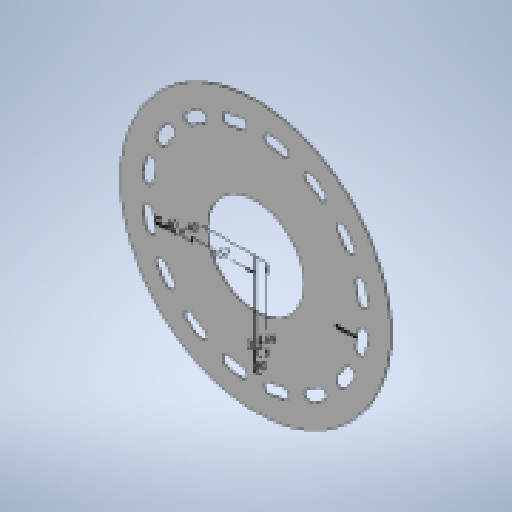
# Autodesk Inventor part: DMF 2.1 01 45 Gear ring 5
Saved by Autodesk Inventor 2026.2 (Build 302298000, 298)
## iProperties
Created: 2024-04-30
Part Number: DMF 2.1 01 45 Gear ring 5
Material: Generic
Document SubType Name: Sheet Metal
Designer: admin
Stock Number: Барабан_Сектор_Усилителя
Density: 1 g/cm^3
Sheet Metal Rule: Default
Sheet Metal Width: 0,000 mm
Sheet Metal Length: 0,000 mm
Sheet Metal Area: 0,000 mm^2
Appearance: Default
Author: pokla
Autodesk Inventor part; units mm, degrees
ref_plane "YZ Plane" through (0, 0, 0) normal (1, 0, 0) x (0, 1, 0)
ref_plane "XZ Plane" through (0, 0, 0) normal (0, 1, 0) x (-1, 0, 0)
ref_plane "XY Plane" through (0, 0, 0) normal (0, 0, 1) x (1, 0, 0)
sketch "Sketch1" plane through (0, 0, 0) normal (0, 0, 1) x (1, 0, 0)
  circle A0 centre (0, 0) radius 100
  circle A1 centre (0, 0) radius 280
  circle A2 centre (0, 0) radius 225 construction
  line L0 (-161.6581, -280) -> (-323.3162, 0)
  line L1 (-323.3162, 0) -> (-161.6581, 280)
  line L2 (-161.6581, 280) -> (161.6581, 280)
  line L3 (161.6581, 280) -> (323.3162, 0)
  line L4 (323.3162, 0) -> (161.6581, -280)
  line L5 (161.6581, -280) -> (-161.6581, -280)
  arc A3 (-28.3948, 223.2011) -> (-59.182, 217.0771) centre (0, 0) ccw construction
  arc A4 (-29.783, 234.1132) -> (-62.0754, 227.6898) centre (0, 0) ccw
  arc A5 (-27.0066, 212.2891) -> (-56.2887, 206.4645) centre (0, 0) ccw
  arc A6 (-27.0066, 212.2891) -> (-29.783, 234.1132) centre (-28.3948, 223.2011) ccw
  arc A7 (-62.0754, 227.6898) -> (-56.2887, 206.4645) centre (-59.182, 217.0771) ccw
  line L6 (-28.3948, 223.2011) -> (0, 0) construction
  line L7 (-59.182, 217.0771) -> (0, 0) construction
  line L8 (0, 0) -> (0, 100) construction
  line L9 (-43.8953, 220.6767) -> (0, 0) construction
  arc A8 (-106.1903, 185.7945) -> (-131.0145, 169.2076) centre (0, 0) ccw
  arc A9 (-106.1903, 185.7945) -> (-117.1071, 204.8949) centre (-111.6487, 195.3447) ccw
  arc A10 (-144.4833, 186.6027) -> (-131.0145, 169.2076) centre (-137.7489, 177.9052) ccw
  arc A11 (-117.1071, 204.8949) -> (-144.4833, 186.6027) centre (0, 0) ccw
  arc A12 (-111.6487, 195.3447) -> (-137.7489, 177.9052) centre (0, 0) ccw construction
  arc A13 (-169.2076, 131.0145) -> (-185.7945, 106.1903) centre (0, 0) ccw
  arc A14 (-169.2076, 131.0145) -> (-186.6027, 144.4833) centre (-177.9052, 137.7489) ccw
  arc A15 (-204.8949, 117.1071) -> (-185.7945, 106.1903) centre (-195.3447, 111.6487) ccw
  arc A16 (-186.6027, 144.4833) -> (-204.8949, 117.1071) centre (0, 0) ccw
  arc A17 (-177.9052, 137.7489) -> (-195.3447, 111.6487) centre (0, 0) ccw construction
  arc A18 (-206.4645, 56.2887) -> (-212.2891, 27.0066) centre (0, 0) ccw
  arc A19 (-206.4645, 56.2887) -> (-227.6898, 62.0754) centre (-217.0771, 59.182) ccw
  arc A20 (-234.1132, 29.783) -> (-212.2891, 27.0066) centre (-223.2011, 28.3948) ccw
  arc A21 (-227.6898, 62.0754) -> (-234.1132, 29.783) centre (0, 0) ccw
  arc A22 (-217.0771, 59.182) -> (-223.2011, 28.3948) centre (0, 0) ccw construction
  arc A23 (-212.2891, -27.0066) -> (-206.4645, -56.2887) centre (0, 0) ccw
  arc A24 (-212.2891, -27.0066) -> (-234.1132, -29.783) centre (-223.2011, -28.3948) ccw
  arc A25 (-227.6898, -62.0754) -> (-206.4645, -56.2887) centre (-217.0771, -59.182) ccw
  arc A26 (-234.1132, -29.783) -> (-227.6898, -62.0754) centre (0, 0) ccw
  arc A27 (-223.2011, -28.3948) -> (-217.0771, -59.182) centre (0, 0) ccw construction
  arc A28 (-185.7945, -106.1903) -> (-169.2076, -131.0145) centre (0, 0) ccw
  arc A29 (-185.7945, -106.1903) -> (-204.8949, -117.1071) centre (-195.3447, -111.6487) ccw
  arc A30 (-186.6027, -144.4833) -> (-169.2076, -131.0145) centre (-177.9052, -137.7489) ccw
  arc A31 (-204.8949, -117.1071) -> (-186.6027, -144.4833) centre (0, 0) ccw
  arc A32 (-195.3447, -111.6487) -> (-177.9052, -137.7489) centre (0, 0) ccw construction
  arc A33 (-131.0145, -169.2076) -> (-106.1903, -185.7945) centre (0, 0) ccw
  arc A34 (-131.0145, -169.2076) -> (-144.4833, -186.6027) centre (-137.7489, -177.9052) ccw
  arc A35 (-117.1071, -204.8949) -> (-106.1903, -185.7945) centre (-111.6487, -195.3447) ccw
  arc A36 (-144.4833, -186.6027) -> (-117.1071, -204.8949) centre (0, 0) ccw
  arc A37 (-137.7489, -177.9052) -> (-111.6487, -195.3447) centre (0, 0) ccw construction
  arc A38 (-56.2887, -206.4645) -> (-27.0066, -212.2891) centre (0, 0) ccw
  arc A39 (-56.2887, -206.4645) -> (-62.0754, -227.6898) centre (-59.182, -217.0771) ccw
  arc A40 (-29.783, -234.1132) -> (-27.0066, -212.2891) centre (-28.3948, -223.2011) ccw
  arc A41 (-62.0754, -227.6898) -> (-29.783, -234.1132) centre (0, 0) ccw
  arc A42 (-59.182, -217.0771) -> (-28.3948, -223.2011) centre (0, 0) ccw construction
  arc A43 (27.0066, -212.2891) -> (56.2887, -206.4645) centre (0, 0) ccw
  arc A44 (27.0066, -212.2891) -> (29.783, -234.1132) centre (28.3948, -223.2011) ccw
  arc A45 (62.0754, -227.6898) -> (56.2887, -206.4645) centre (59.182, -217.0771) ccw
  arc A46 (29.783, -234.1132) -> (62.0754, -227.6898) centre (0, 0) ccw
  arc A47 (28.3948, -223.2011) -> (59.182, -217.0771) centre (0, 0) ccw construction
  arc A48 (106.1903, -185.7945) -> (131.0145, -169.2076) centre (0, 0) ccw
  arc A49 (106.1903, -185.7945) -> (117.1071, -204.8949) centre (111.6487, -195.3447) ccw
  arc A50 (144.4833, -186.6027) -> (131.0145, -169.2076) centre (137.7489, -177.9052) ccw
  arc A51 (117.1071, -204.8949) -> (144.4833, -186.6027) centre (0, 0) ccw
  arc A52 (111.6487, -195.3447) -> (137.7489, -177.9052) centre (0, 0) ccw construction
  arc A53 (169.2076, -131.0145) -> (185.7945, -106.1903) centre (0, 0) ccw
  arc A54 (169.2076, -131.0145) -> (186.6027, -144.4833) centre (177.9052, -137.7489) ccw
  arc A55 (204.8949, -117.1071) -> (185.7945, -106.1903) centre (195.3447, -111.6487) ccw
  arc A56 (186.6027, -144.4833) -> (204.8949, -117.1071) centre (0, 0) ccw
  arc A57 (177.9052, -137.7489) -> (195.3447, -111.6487) centre (0, 0) ccw construction
  arc A58 (206.4645, -56.2887) -> (212.2891, -27.0066) centre (0, 0) ccw
  arc A59 (206.4645, -56.2887) -> (227.6898, -62.0754) centre (217.0771, -59.182) ccw
  arc A60 (234.1132, -29.783) -> (212.2891, -27.0066) centre (223.2011, -28.3948) ccw
  arc A61 (227.6898, -62.0754) -> (234.1132, -29.783) centre (0, 0) ccw
  arc A62 (217.0771, -59.182) -> (223.2011, -28.3948) centre (0, 0) ccw construction
  arc A63 (212.2891, 27.0066) -> (206.4645, 56.2887) centre (0, 0) ccw
  arc A64 (212.2891, 27.0066) -> (234.1132, 29.783) centre (223.2011, 28.3948) ccw
  arc A65 (227.6898, 62.0754) -> (206.4645, 56.2887) centre (217.0771, 59.182) ccw
  arc A66 (234.1132, 29.783) -> (227.6898, 62.0754) centre (0, 0) ccw
  arc A67 (223.2011, 28.3948) -> (217.0771, 59.182) centre (0, 0) ccw construction
  arc A68 (185.7945, 106.1903) -> (169.2076, 131.0145) centre (0, 0) ccw
  arc A69 (185.7945, 106.1903) -> (204.8949, 117.1071) centre (195.3447, 111.6487) ccw
  arc A70 (186.6027, 144.4833) -> (169.2076, 131.0145) centre (177.9052, 137.7489) ccw
  arc A71 (204.8949, 117.1071) -> (186.6027, 144.4833) centre (0, 0) ccw
  arc A72 (195.3447, 111.6487) -> (177.9052, 137.7489) centre (0, 0) ccw construction
  arc A73 (131.0145, 169.2076) -> (106.1903, 185.7945) centre (0, 0) ccw
  arc A74 (131.0145, 169.2076) -> (144.4833, 186.6027) centre (137.7489, 177.9052) ccw
  arc A75 (117.1071, 204.8949) -> (106.1903, 185.7945) centre (111.6487, 195.3447) ccw
  arc A76 (144.4833, 186.6027) -> (117.1071, 204.8949) centre (0, 0) ccw
  arc A77 (137.7489, 177.9052) -> (111.6487, 195.3447) centre (0, 0) ccw construction
  arc A78 (56.2887, 206.4645) -> (27.0066, 212.2891) centre (0, 0) ccw
  arc A79 (56.2887, 206.4645) -> (62.0754, 227.6898) centre (59.182, 217.0771) ccw
  arc A80 (29.783, 234.1132) -> (27.0066, 212.2891) centre (28.3948, 223.2011) ccw
  arc A81 (62.0754, 227.6898) -> (29.783, 234.1132) centre (0, 0) ccw
  arc A82 (59.182, 217.0771) -> (28.3948, 223.2011) centre (0, 0) ccw construction
  point P0 (0, -280)
  point P1 (242.4871, 140)
  point P2 (-242.4871, 140)
  point P3 (-125.0033, 187.0807)
  point P4 (-187.0807, 125.0033)
  point P5 (-220.6767, 43.8953)
  point P6 (-220.6767, -43.8953)
  point P7 (-187.0807, -125.0033)
  point P8 (-125.0033, -187.0807)
  point P9 (-43.8953, -220.6767)
  point P10 (43.8953, -220.6767)
  point P11 (125.0033, -187.0807)
  point P12 (187.0807, -125.0033)
  point P13 (220.6767, -43.8953)
  point P14 (220.6767, 43.8953)
  point P15 (187.0807, 125.0033)
  point P16 (125.0033, 187.0807)
  point P17 (43.8953, 220.6767)
  dimension "d31" = 560
  dimension "d32" = 200
  dimension "d39" = 450
  dimension "d56" = 11
  dimension "d57" = 8
  dimension "d58" = 11.25
  dimension "d61" = 360
  measures "d56" radius of A7
  measures "d57" angle of L7 L6
  measures "d58" angle of L8 L9
extrude "Plate4" add sketch "Sketch1" along normal blind 2 contours A1
sketch "Sketch5" plane through (0, 0, 2) normal (0, 0, 1) x (1, 0, 0)
  line L0 (-1.6, -169) -> (1.6, -169)
  line L1 (1.6, -169) -> (1.6, -209)
  line L2 (1.6, -209) -> (-1.6, -209)
  line L3 (-1.6, -209) -> (-1.6, -169)
  line L4 (-207, -40) -> (-167, -40)
  line L5 (-167, -40) -> (-167, -43.2)
  line L6 (-167, -43.2) -> (-207, -43.2)
  line L7 (-207, -43.2) -> (-207, -40)
  line L8 (0, 0) -> (0, -169)
  line L9 (167, -40) -> (207, -40)
  line L10 (207, -40) -> (207, -43.2)
  line L11 (207, -43.2) -> (167, -43.2)
  line L12 (167, -43.2) -> (167, -40)
  dimension "d74" = 3.2
  dimension "d75" = 40
  dimension "d76" = 40
  dimension "d77" = 40
  dimension "d78" = 167
  dimension "d79" = 169
  constraints: 26 end point, 6 parallel, 3 equal length, 3 horizontal, 3 perpendicular, 1 collinear, 1 midpoint, 1 vertical, 1 other
  measures "d74" distance of L0.start L0.end
  measures "d75" distance of L0.end L1.end
  measures "d76" distance of L4.start L4.end
  measures "d77" distance from line of L8.start L4
  measures "d78" distance between parallel lines of L8 L5
  measures "d79" distance from line of L0 L8.start
mark "Mark1"
equation "\"d31\" = Колесо_диам3_борт_ступицы"
equation "\"d63\" = Thickness"
equation "\"BendRadius\" = Thickness"
equation "\"BendReliefWidth\" = Thickness"
equation "\"BendReliefDepth\" = 0.5 * Thickness"
equation "\"CornerReliefSize\" = 4 * Thickness"
equation "\"MinimumRemnant\" = 2 * Thickness"
equation "\"TransitionRadius\" = BendRadius"
equation "\"JacobiRadiusSize\" = BendRadius"
equation "\"GapSize\" = Thickness"
equation "\"Колесо_диам3_борт_ступицы\" = 560"
equation "\"Thickness\" = 2"
body "Solid3"
